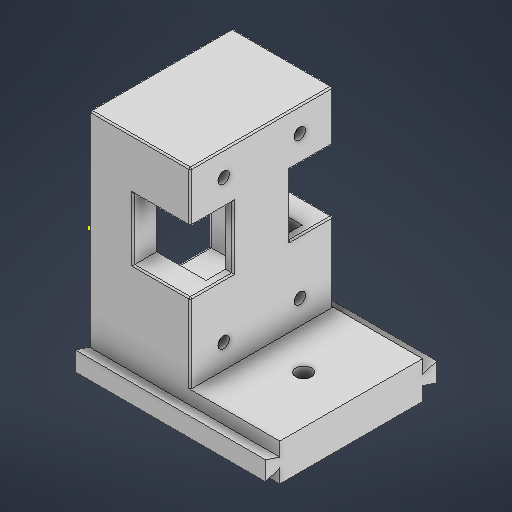
# Autodesk Inventor part: motorHousingStraight
Saved by Autodesk Inventor 2026 (Build 300175000, 175)
## iProperties
Created: 2025-04-17
Part Number: motorHousingStraight
Material: Generic
Document SubType Name: Modeling
Designer: Elizabeth
Density: 1 g/cm^3
Appearance: Default
Author: Elizabeth
Autodesk Inventor part; units mm, degrees
ref_plane "YZ Plane" through (0, 0, 0) normal (1, 0, 0) x (0, 1, 0)
ref_plane "XZ Plane" through (0, 0, 0) normal (0, 1, 0) x (-1, 0, 0)
ref_plane "XY Plane" through (0, 0, 0) normal (0, 0, 1) x (1, 0, 0)
sketch "Sketch1" plane through (0, 0, 0) normal (0, 0, 1) x (1, 0, 0)
  line L0 (-20.0425, -15.7111) -> (9.4023, 1.2889) construction
  line L1 (-1.8425, 18.3873) -> (-20.0425, 18.3873)
  line L2 (-20.0425, 18.3873) -> (-20.0425, -18.8127)
  line L3 (-20.0425, -15.8127) -> (-1.8425, -15.8127)
  line L4 (-1.8425, -15.8127) -> (-1.8425, 18.3873)
  line L5 (-20.0425, 18.3873) -> (-20.0425, 21.3873)
  line L6 (-20.0425, 18.3873) -> (-17.4444, 19.8873) construction
  line L7 (-20.0425, 21.3873) -> (1.1575, 21.3873)
  line L8 (1.1575, 21.3873) -> (1.1575, -18.8127)
  line L9 (1.1575, -18.8127) -> (-20.0425, -18.8127)
  line L10 (-20.0425, -15.8127) -> (-1.856, -5.3127) construction
  line L11 (-20.0425, -26.6146) -> (19.9575, -26.6146)
  line L12 (19.9575, -26.6146) -> (19.9575, -18.8127)
  line L13 (-20.0425, -26.6146) -> (-20.0425, -18.8127)
  line L14 (19.9575, -18.8127) -> (1.1575, -18.8127)
  point P0 (-20.0425, -18.8127)
  constraints: 30 end point, 5 perpendicular, 2 point on line, 1 equal length, 1 horizontal, 1 vertical
extrude "Extrusion1" add sketch "Sketch1" against normal blind 30
sketch "Sketch2" plane through (-20.0425, -26.6146, 0) normal (-1, 0, 0) x (0, 0, 1)
  line L0 (0, 48.0019) -> (-30, 48.0019) projected
  line L1 (0, 7.8019) -> (-30, 7.8019) projected
  line L2 (0, 48.0019) -> (0, 0) projected
  line L3 (-4.9, 45.2019) -> (-4.9, 10.7019)
  line L4 (-25.1, 10.7019) -> (-25.1, 45.2019)
  line L5 (-7, 42.9019) -> (-23, 42.9019)
  line L6 (-23, 42.9019) -> (-23, 12.9019)
  line L7 (-23, 12.9019) -> (-7, 12.9019)
  line L8 (-7, 12.9019) -> (-7, 42.9019)
  circle A0 centre (-23, 42.9019) radius 1.2
  circle A1 centre (-7, 42.9019) radius 1.2
  circle A2 centre (-23, 12.9019) radius 1.2
  circle A3 centre (-7, 12.9019) radius 1.2
  line L9 (-30, 4.901) -> (-30, 2.901)
  line L10 (-30, 2.901) -> (-30, 3.901)
  line L11 (-33, 5.901) -> (-30, 4.901)
  line L12 (-33, 1.901) -> (-30, 2.901)
  line L13 (-33, 1.901) -> (-33, 5.901)
  line L14 (0, 4.901) -> (0, 2.901)
  line L15 (0, 2.901) -> (0, 3.901)
  line L16 (3, 5.901) -> (0, 4.901)
  line L17 (3, 1.901) -> (0, 2.901)
  line L18 (3, 1.901) -> (3, 5.901)
  line L19 (-7, 10.7019) -> (-6.5971, 10.7019)
  line L20 (-25.1, 45.2019) -> (-4.9, 45.2019)
  line L21 (-4.9, 10.7019) -> (-25.1, 10.7019)
  point P0 (0, 26.6146)
  point P1 (-25.1, 45.0019)
  point P2 (-4.9, 10.8019)
  point P3 (-25.1, 10.8019)
  point P4 (-4.9, 45.1019)
  point P5 (-25.1, 45.1019)
  dimension "d21" = 2.4
  dimension "d22" = 2.4
  dimension "d23" = 2.4
  dimension "d24" = 2.4
  constraints: 38 end point, 7 point on line, 4 centre point, 4 coincident, 3 parallel, 2 midpoint, 1 perpendicular, 1 vertical
  measures "d21" diameter of A0
  measures "d22" diameter of A1
  measures "d23" diameter of A2
  measures "d24" diameter of A3
extrude "Extrusion2" cut sketch "Sketch2" against normal blind 19.6 contours L3 L21 L19 L4 L20 | A0 L6 L5 | L5 L6 A0 | L5 A1 L8 A3 L7 A2 L6 A0 | A1 L8 L5 | L5 L8 A1 | A2 L7 L6 | L6 L7 A2 | A3 L7 L8 | L8 L7 A3
sketch "Sketch3" plane through (1.1575, -18.8127, 0) normal (1, 0, 0) x (0, 0, -1)
  line L0 (0, 16.6) -> (0, 29.6)
  line L1 (0, 16.6) -> (9, 16.6)
  line L2 (9, 16.6) -> (9, 29.6)
  line L3 (9, 29.6) -> (0, 29.6)
  line L4 (30, 16.6) -> (30, 29.6)
  line L5 (30, 16.6) -> (21, 16.6)
  line L6 (21, 16.6) -> (21, 29.6)
  line L7 (21, 29.6) -> (30, 29.6)
  line L8 (30, 40.2) -> (0, 40.2)
  line L9 (25.1, 38.7) -> (4.9, 38.7)
  line L10 (25.1, 4.5) -> (25.1, 38.7)
  point P0 (0, 18.8127)
  dimension "d14" = 12
  dimension "d15" = 13
  dimension "d16" = 9.1
  dimension "d17" = 4.1
  constraints: 22 end point, 2 perpendicular, 1 horizontal
  measures "d14" distance between parallel lines of L6 L2
  measures "d15" distance of L5.end L6.end
  measures "d16" distance between parallel lines of L7 L9
  measures "d17" distance between parallel lines of L6 L10
extrude "Extrusion3" cut sketch "Sketch3" against normal blind 12
extrude "Extrusion4" cut sketch "Sketch2" against normal blind 21.2 contours A0 L6 L5 | L5 L6 A0 | A1 L8 L5 | L5 L8 A1 | A2 L7 L6 | L6 L7 A2 | A3 L7 L8 | L8 L7 A3
sketch "Sketch4" plane through (-20.0425, -26.6146, 0) normal (-1, 0, 0) x (0, 0, 1)
  point P0 (0, 26.6146)
extrude "Extrusion5" add sketch "Sketch2" against normal blind 40 contours L16 L18 L17 L2 | L9 L12 L13 L11
sketch "Sketch5" plane through (-20.0425, -26.6146, 0) normal (0, -1, 0) x (1, 0, 0)
  line L0 (40, -15) -> (30, -15)
  circle A0 centre (30, -15) radius 1.65
  point P0 (20.0425, 0)
  dimension "d29" = 10
  dimension "d30" = 3.3
  constraints: 2 end point, 1 centre point, 1 coincident, 1 horizontal
  measures "d29" distance of L0.start L0.end
  measures "d30" diameter of A0
extrude "Extrusion6" cut sketch "Sketch5" against normal blind 7.802
fillet "Fillet1" radius 0.3 22 edges at (-4.8425, 10.7873, -30) (1.1575, 16.0873, -30) (1.1575, 4.2873, -21) (1.1575, -2.2127, -25.5) (1.1575, 10.7873, -25.5) (-4.8425, -2.2127, -30) (-10.8425, 4.2873, -30) (1.1575, -10.5127, -30) (1.1575, -10.5127, 0) (1.1575, -2.2127, -4.5) (1.1575, 4.2873, -9) (-4.8425, -2.2127, 0) (1.1575, 10.7873, -4.5) (1.1575, 16.0873, 0) (1.1575, 21.3873, -15) (-9.4425, 21.3873, 0) (-9.4425, 21.3873, -30) (-20.0425, 21.3873, -15) (-20.0425, -0.1632, -30) (-20.0425, -0.1632, 0) (-10.8425, 4.2873, 0) (-4.8425, 10.7873, 0)
fillet "Fillet2" radius 0.5 4 edges at (-20.0425, 1.3373, -25.1) (-20.0425, 1.3373, -4.9) (-20.0425, 18.5873, -15) (-20.0425, -15.9127, -15)
body "Solid1"
